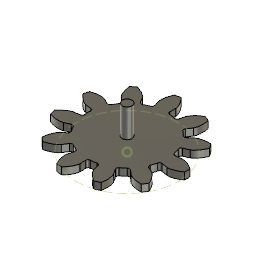
Slave gear (Autodesk Fusion 360 design; units mm, degrees)
description: Spur Gear; Module: 6.55; Num Teeth: 11; Pressure Angle: 20.0; Backlash: 0.00 mm
Autodesk Fusion 360 part; units mm, degrees
(part 1 of 3)
sketch "Sketch1" plane through (0, 0, 0) normal (0, 0, 1) x (1, 0, 0) in component "Spur Gear (11 teeth)"
  circle A0 centre (0, 0) radius 28.1142
extrude "Extrude1" add sketch "Sketch1" along normal blind 10 in component "Spur Gear (11 teeth)"
sketch "Sketch2" plane through (0, 0, 0) normal (0, 0, 1) x (1, 0, 0) in component "Spur Gear (11 teeth)"
  spline S0 degree 5 poles (33.4323, -5.3166) (33.4583, -5.3207) (33.5104, -5.3281) (33.5887, -5.3365) (33.6936, -5.3428) (33.8252, -5.344) (33.9572, -5.3403) (34.0895, -5.3337) (34.2219, -5.3256) (34.3544, -5.3164) (34.4869, -5.3059) (34.6196, -5.2938) (34.7523, -5.2796) (34.8851, -5.263) (35.018, -5.2439) (35.1509, -5.2227) (35.2838, -5.1996) (35.4168, -5.175) (35.5497, -5.149) (35.6826, -5.1217) (35.8155, -5.093) (35.9483, -5.0629) (36.0811, -5.0314) (36.2138, -4.9983) (36.3465, -4.9637) (36.4791, -4.9277) (36.6117, -4.8903) (36.7441, -4.8516) (36.8765, -4.8117) (37.0087, -4.7706) (37.1408, -4.7282) (37.2729, -4.6847) (37.4048, -4.6398) (37.5366, -4.5938) (37.6683, -4.5466) (37.7998, -4.4982) (37.9312, -4.4486) (38.0624, -4.3979) (38.1935, -4.3461) (38.3245, -4.2932) (38.4553, -4.2392) (38.5859, -4.1841) (38.7163, -4.1279) (38.8466, -4.0706) (38.9767, -4.0123) (39.1066, -3.9529) (39.2363, -3.8924) (39.3658, -3.831) (39.4951, -3.7685) (39.6243, -3.705) (39.7532, -3.6406) (39.8819, -3.5751) (40.0104, -3.5086) (40.1386, -3.4412) (40.2667, -3.3727) (40.3945, -3.3033) (40.5221, -3.233) (40.6494, -3.1617) (40.7765, -3.0895) (40.9034, -3.0163) (41.03, -2.9422) (41.1564, -2.8672) (41.2825, -2.7912) (41.4084, -2.7144) (41.534, -2.6366) (41.6593, -2.558) (41.7844, -2.4784) (41.9092, -2.398) (42.0337, -2.3167) (42.1579, -2.2345) (42.2818, -2.1514) (42.3808, -2.0843) (42.4548, -2.0335) (42.5042, -1.9995) (42.5288, -1.9825) knots 0 0 0 0 0 0 0.01428571 0.02857143 0.04285714 0.05714286 0.07142857 0.08571429 0.1 0.11428571 0.12857143 0.14285714 0.15714286 0.17142857 0.18571429 0.2 0.21428571 0.22857143 0.24285714 0.25714286 0.27142857 0.28571429 0.3 0.31428571 0.32857143 0.34285714 0.35714286 0.37142857 0.38571429 0.4 0.41428571 0.42857143 0.44285714 0.45714286 0.47142857 0.48571429 0.5 0.51428571 0.52857143 0.54285714 0.55714286 0.57142857 0.58571429 0.6 0.61428571 0.62857143 0.64285714 0.65714286 0.67142857 0.68571429 0.7 0.71428571 0.72857143 0.74285714 0.75714286 0.77142857 0.78571429 0.8 0.81428571 0.82857143 0.84285714 0.85714286 0.87142857 0.88571429 0.9 0.91428571 0.92857143 0.94285714 0.95714286 0.97142857 0.98571429 1 1 1 1 1 1
  spline S1 degree 5 poles (33.4323, 5.3166) (33.4583, 5.3207) (33.5104, 5.3281) (33.5887, 5.3365) (33.6936, 5.3428) (33.8252, 5.344) (33.9572, 5.3403) (34.0895, 5.3337) (34.2219, 5.3256) (34.3544, 5.3164) (34.4869, 5.3059) (34.6196, 5.2938) (34.7523, 5.2796) (34.8851, 5.263) (35.018, 5.2439) (35.1509, 5.2227) (35.2838, 5.1996) (35.4168, 5.175) (35.5497, 5.149) (35.6826, 5.1217) (35.8155, 5.093) (35.9483, 5.0629) (36.0811, 5.0314) (36.2138, 4.9983) (36.3465, 4.9637) (36.4791, 4.9277) (36.6117, 4.8903) (36.7441, 4.8516) (36.8765, 4.8117) (37.0087, 4.7706) (37.1408, 4.7282) (37.2729, 4.6847) (37.4048, 4.6398) (37.5366, 4.5938) (37.6683, 4.5466) (37.7998, 4.4982) (37.9312, 4.4486) (38.0624, 4.3979) (38.1935, 4.3461) (38.3245, 4.2932) (38.4553, 4.2392) (38.5859, 4.1841) (38.7163, 4.1279) (38.8466, 4.0706) (38.9767, 4.0123) (39.1066, 3.9529) (39.2363, 3.8924) (39.3658, 3.831) (39.4951, 3.7685) (39.6243, 3.705) (39.7532, 3.6406) (39.8819, 3.5751) (40.0104, 3.5086) (40.1386, 3.4412) (40.2667, 3.3727) (40.3945, 3.3033) (40.5221, 3.233) (40.6494, 3.1617) (40.7765, 3.0895) (40.9034, 3.0163) (41.03, 2.9422) (41.1564, 2.8672) (41.2825, 2.7912) (41.4084, 2.7144) (41.534, 2.6366) (41.6593, 2.558) (41.7844, 2.4784) (41.9092, 2.398) (42.0337, 2.3167) (42.1579, 2.2345) (42.2818, 2.1514) (42.3808, 2.0843) (42.4548, 2.0335) (42.5042, 1.9995) (42.5288, 1.9825) knots 0 0 0 0 0 0 0.01428571 0.02857143 0.04285714 0.05714286 0.07142857 0.08571429 0.1 0.11428571 0.12857143 0.14285714 0.15714286 0.17142857 0.18571429 0.2 0.21428571 0.22857143 0.24285714 0.25714286 0.27142857 0.28571429 0.3 0.31428571 0.32857143 0.34285714 0.35714286 0.37142857 0.38571429 0.4 0.41428571 0.42857143 0.44285714 0.45714286 0.47142857 0.48571429 0.5 0.51428571 0.52857143 0.54285714 0.55714286 0.57142857 0.58571429 0.6 0.61428571 0.62857143 0.64285714 0.65714286 0.67142857 0.68571429 0.7 0.71428571 0.72857143 0.74285714 0.75714286 0.77142857 0.78571429 0.8 0.81428571 0.82857143 0.84285714 0.85714286 0.87142857 0.88571429 0.9 0.91428571 0.92857143 0.94285714 0.95714286 0.97142857 0.98571429 1 1 1 1 1 1
  arc A0 (42.5288, -1.9825) -> (42.5288, 1.9825) centre (0, 0) ccw
  line L0 (27.7554, -4.4154) -> (33.4323, -5.3166)
  line L1 (27.7554, 4.4154) -> (33.4323, 5.3166)
  line L2 (27.7554, -4.4154) -> (27.7554, 4.4154)
  point P0 (34.0602, -5.3349)
  point P1 (34.6983, -5.2851)
  point P2 (35.3427, -5.1885)
  point P3 (35.9917, -5.0524)
  point P4 (36.644, -4.8806)
  point P5 (37.2988, -4.6757)
  point P6 (37.955, -4.4392)
  point P7 (38.612, -4.1726)
  point P8 (39.2689, -3.8768)
  point P9 (39.9251, -3.5526)
  point P10 (40.5799, -3.2005)
  point P11 (41.2325, -2.8212)
  point P12 (41.8824, -2.4151)
  point P13 (34.0602, 5.3349)
  point P14 (34.6983, 5.2851)
  point P15 (35.3427, 5.1885)
  point P16 (35.9917, 5.0524)
  point P17 (36.644, 4.8806)
  point P18 (37.2988, 4.6757)
  point P19 (37.955, 4.4392)
  point P20 (38.612, 4.1726)
  point P21 (39.2689, 3.8768)
  point P22 (39.9251, 3.5526)
  point P23 (40.5799, 3.2005)
  point P24 (41.2325, 2.8212)
  point P25 (41.8824, 2.4151)
extrude "Extrude2" add sketch "Sketch2" along normal blind 10 in component "Spur Gear (11 teeth)"
fillet "Fillet1" radius 1.5875 2 edges at (27.7651, -4.4169, 5) (27.7651, 4.4169, 5) in component "Spur Gear (11 teeth)"
pattern_circular "C-Pattern1" count 11 over 360 about axis through (0, 0, 0) along (0, 0, 1) of "Extrude2", "Fillet1" in component "Spur Gear (11 teeth)"
sketch "Sketch3" plane through (0, 0, 0) normal (0, 0, 1) x (1, 0, 0) in component "Spur Gear (11 teeth)"
  circle A0 centre (0, 0) radius 36.025 construction
sketch "Sketch1 (2)" plane through (0, 0, 10) normal (0, 0, 1) x (-1, 0, 0)
  arc A0 (-26.3122, 9.9035) -> (-27.4894, 5.8941) centre (0, 0) ccw
  arc A1 (-29.2905, 4.6591) -> (-27.4894, 5.8941) centre (-29.0416, 6.2269) ccw
  line L0 (-29.2905, 4.6591) -> (-33.4323, 5.3166)
  spline S0 degree 5 poles (-33.4323, 5.3166) (-33.4583, 5.3207) (-33.5104, 5.3281) (-33.5887, 5.3365) (-33.6936, 5.3428) (-33.8252, 5.344) (-33.9572, 5.3403) (-34.0895, 5.3337) (-34.2219, 5.3256) (-34.3544, 5.3164) (-34.4869, 5.3059) (-34.6196, 5.2938) (-34.7523, 5.2796) (-34.8851, 5.263) (-35.018, 5.2439) (-35.1509, 5.2227) (-35.2838, 5.1996) (-35.4168, 5.175) (-35.5497, 5.149) (-35.6826, 5.1217) (-35.8155, 5.093) (-35.9483, 5.0629) (-36.0811, 5.0314) (-36.2138, 4.9983) (-36.3465, 4.9637) (-36.4791, 4.9277) (-36.6117, 4.8903) (-36.7441, 4.8516) (-36.8765, 4.8117) (-37.0087, 4.7706) (-37.1408, 4.7282) (-37.2729, 4.6847) (-37.4048, 4.6398) (-37.5366, 4.5938) (-37.6683, 4.5466) (-37.7998, 4.4982) (-37.9312, 4.4486) (-38.0624, 4.3979) (-38.1935, 4.3461) (-38.3245, 4.2932) (-38.4553, 4.2392) (-38.5859, 4.1841) (-38.7163, 4.1279) (-38.8466, 4.0706) (-38.9767, 4.0123) (-39.1066, 3.9529) (-39.2363, 3.8924) (-39.3658, 3.831) (-39.4951, 3.7685) (-39.6243, 3.705) (-39.7532, 3.6406) (-39.8819, 3.5751) (-40.0104, 3.5086) (-40.1386, 3.4412) (-40.2667, 3.3727) (-40.3945, 3.3033) (-40.5221, 3.233) (-40.6494, 3.1617) (-40.7765, 3.0895) (-40.9034, 3.0163) (-41.03, 2.9422) (-41.1564, 2.8672) (-41.2825, 2.7912) (-41.4084, 2.7144) (-41.534, 2.6366) (-41.6593, 2.558) (-41.7844, 2.4784) (-41.9092, 2.398) (-42.0337, 2.3167) (-42.1579, 2.2345) (-42.2818, 2.1514) (-42.3808, 2.0843) (-42.4548, 2.0335) (-42.5042, 1.9995) (-42.5288, 1.9825) knots 0 0 0 0 0 0 0.01428571 0.02857143 0.04285714 0.05714286 0.07142857 0.08571429 0.1 0.11428571 0.12857143 0.14285714 0.15714286 0.17142857 0.18571429 0.2 0.21428571 0.22857143 0.24285714 0.25714286 0.27142857 0.28571429 0.3 0.31428571 0.32857143 0.34285714 0.35714286 0.37142857 0.38571429 0.4 0.41428571 0.42857143 0.44285714 0.45714286 0.47142857 0.48571429 0.5 0.51428571 0.52857143 0.54285714 0.55714286 0.57142857 0.58571429 0.6 0.61428571 0.62857143 0.64285714 0.65714286 0.67142857 0.68571429 0.7 0.71428571 0.72857143 0.74285714 0.75714286 0.77142857 0.78571429 0.8 0.81428571 0.82857143 0.84285714 0.85714286 0.87142857 0.88571429 0.9 0.91428571 0.92857143 0.94285714 0.95714286 0.97142857 0.98571429 1 1 1 1 1 1
  arc A2 (-42.5288, 1.9825) -> (-42.5288, -1.9825) centre (0, 0) ccw
  spline S1 degree 5 poles (-42.5288, -1.9825) (-42.5042, -1.9995) (-42.4548, -2.0335) (-42.3808, -2.0843) (-42.2818, -2.1514) (-42.1579, -2.2345) (-42.0337, -2.3167) (-41.9092, -2.398) (-41.7844, -2.4784) (-41.6593, -2.558) (-41.534, -2.6366) (-41.4084, -2.7144) (-41.2825, -2.7912) (-41.1564, -2.8672) (-41.03, -2.9422) (-40.9034, -3.0163) (-40.7765, -3.0895) (-40.6494, -3.1617) (-40.5221, -3.233) (-40.3945, -3.3033) (-40.2667, -3.3727) (-40.1386, -3.4412) (-40.0104, -3.5086) (-39.8819, -3.5751) (-39.7532, -3.6406) (-39.6243, -3.705) (-39.4951, -3.7685) (-39.3658, -3.831) (-39.2363, -3.8924) (-39.1066, -3.9529) (-38.9767, -4.0123) (-38.8466, -4.0706) (-38.7163, -4.1279) (-38.5859, -4.1841) (-38.4553, -4.2392) (-38.3245, -4.2932) (-38.1935, -4.3461) (-38.0624, -4.3979) (-37.9312, -4.4486) (-37.7998, -4.4982) (-37.6683, -4.5466) (-37.5366, -4.5938) (-37.4048, -4.6398) (-37.2729, -4.6847) (-37.1408, -4.7282) (-37.0087, -4.7706) (-36.8765, -4.8117) (-36.7441, -4.8516) (-36.6117, -4.8903) (-36.4791, -4.9277) (-36.3465, -4.9637) (-36.2138, -4.9983) (-36.0811, -5.0314) (-35.9483, -5.0629) (-35.8155, -5.093) (-35.6826, -5.1217) (-35.5497, -5.149) (-35.4168, -5.175) (-35.2838, -5.1996) (-35.1509, -5.2227) (-35.018, -5.2439) (-34.8851, -5.263) (-34.7523, -5.2796) (-34.6196, -5.2938) (-34.4869, -5.3059) (-34.3544, -5.3164) (-34.2219, -5.3256) (-34.0895, -5.3337) (-33.9572, -5.3403) (-33.8252, -5.344) (-33.6936, -5.3428) (-33.5887, -5.3365) (-33.5104, -5.3281) (-33.4583, -5.3207) (-33.4323, -5.3166) knots -1 -1 -1 -1 -1 -1 -0.98571429 -0.97142857 -0.95714286 -0.94285714 -0.92857143 -0.91428571 -0.9 -0.88571429 -0.87142857 -0.85714286 -0.84285714 -0.82857143 -0.81428571 -0.8 -0.78571429 -0.77142857 -0.75714286 -0.74285714 -0.72857143 -0.71428571 -0.7 -0.68571429 -0.67142857 -0.65714286 -0.64285714 -0.62857143 -0.61428571 -0.6 -0.58571429 -0.57142857 -0.55714286 -0.54285714 -0.52857143 -0.51428571 -0.5 -0.48571429 -0.47142857 -0.45714286 -0.44285714 -0.42857143 -0.41428571 -0.4 -0.38571429 -0.37142857 -0.35714286 -0.34285714 -0.32857143 -0.31428571 -0.3 -0.28571429 -0.27142857 -0.25714286 -0.24285714 -0.22857143 -0.21428571 -0.2 -0.18571429 -0.17142857 -0.15714286 -0.14285714 -0.12857143 -0.11428571 -0.1 -0.08571429 -0.07142857 -0.05714286 -0.04285714 -0.02857143 -0.01428571 0 0 0 0 0 0
  line L1 (-33.4323, -5.3166) -> (-29.2905, -4.6591)
  arc A3 (-27.4894, -5.8941) -> (-29.2905, -4.6591) centre (-29.0416, -6.2269) ccw
  arc A4 (-27.4894, -5.8941) -> (-26.3122, -9.9035) centre (0, 0) ccw
  arc A5 (-27.1596, -11.9162) -> (-26.3122, -9.9035) centre (-27.7979, -10.4627) ccw
  line L2 (-27.1596, -11.9162) -> (-30.9994, -13.6023)
  spline S2 degree 5 poles (-30.9994, -13.6023) (-31.0235, -13.6129) (-31.0713, -13.6348) (-31.1418, -13.6701) (-31.2334, -13.7214) (-31.3447, -13.7916) (-31.4538, -13.8661) (-31.5615, -13.9431) (-31.6685, -14.0216) (-31.775, -14.101) (-31.8808, -14.1814) (-31.9859, -14.2633) (-32.0898, -14.347) (-32.1926, -14.4328) (-32.2941, -14.5207) (-32.3944, -14.6104) (-32.4938, -14.7017) (-32.5923, -14.7943) (-32.6901, -14.888) (-32.7871, -14.9829) (-32.8834, -15.0788) (-32.9789, -15.1759) (-33.0735, -15.2743) (-33.1673, -15.3739) (-33.2602, -15.4747) (-33.3523, -15.5767) (-33.4436, -15.6798) (-33.5341, -15.7839) (-33.6239, -15.889) (-33.7129, -15.9951) (-33.8011, -16.1022) (-33.8887, -16.2103) (-33.9754, -16.3193) (-34.0614, -16.4292) (-34.1466, -16.5402) (-34.2311, -16.652) (-34.3149, -16.7647) (-34.3979, -16.8783) (-34.4801, -16.9928) (-34.5617, -17.1081) (-34.6425, -17.2243) (-34.7226, -17.3412) (-34.8019, -17.459) (-34.8805, -17.5777) (-34.9585, -17.6971) (-35.0356, -17.8172) (-35.1121, -17.9382) (-35.1878, -18.0599) (-35.2628, -18.1824) (-35.3371, -18.3056) (-35.4107, -18.4296) (-35.4836, -18.5542) (-35.5558, -18.6796) (-35.6272, -18.8057) (-35.6979, -18.9325) (-35.7679, -19.06) (-35.8372, -19.1881) (-35.9058, -19.3169) (-35.9737, -19.4464) (-36.0409, -19.5766) (-36.1073, -19.7074) (-36.1731, -19.8388) (-36.2381, -19.9709) (-36.3025, -20.1036) (-36.3661, -20.2369) (-36.429, -20.3708) (-36.4912, -20.5054) (-36.5527, -20.6405) (-36.6135, -20.7762) (-36.6735, -20.9125) (-36.7329, -21.0494) (-36.7798, -21.1594) (-36.8147, -21.2421) (-36.8378, -21.2974) (-36.8493, -21.325) knots 0 0 0 0 0 0 0.01428571 0.02857143 0.04285714 0.05714286 0.07142857 0.08571429 0.1 0.11428571 0.12857143 0.14285714 0.15714286 0.17142857 0.18571429 0.2 0.21428571 0.22857143 0.24285714 0.25714286 0.27142857 0.28571429 0.3 0.31428571 0.32857143 0.34285714 0.35714286 0.37142857 0.38571429 0.4 0.41428571 0.42857143 0.44285714 0.45714286 0.47142857 0.48571429 0.5 0.51428571 0.52857143 0.54285714 0.55714286 0.57142857 0.58571429 0.6 0.61428571 0.62857143 0.64285714 0.65714286 0.67142857 0.68571429 0.7 0.71428571 0.72857143 0.74285714 0.75714286 0.77142857 0.78571429 0.8 0.81428571 0.82857143 0.84285714 0.85714286 0.87142857 0.88571429 0.9 0.91428571 0.92857143 0.94285714 0.95714286 0.97142857 0.98571429 1 1 1 1 1 1
  arc A6 (-36.8493, -21.325) -> (-34.7057, -24.6606) centre (0, 0) ccw
  spline S3 degree 5 poles (-34.7057, -24.6606) (-34.6758, -24.6616) (-34.6159, -24.6635) (-34.5261, -24.6662) (-34.4066, -24.6692) (-34.2574, -24.672) (-34.1085, -24.674) (-33.9598, -24.6751) (-33.8113, -24.6753) (-33.6631, -24.6746) (-33.5151, -24.673) (-33.3674, -24.6705) (-33.22, -24.6672) (-33.0729, -24.6629) (-32.926, -24.6576) (-32.7794, -24.6515) (-32.6331, -24.6445) (-32.4871, -24.6365) (-32.3415, -24.6277) (-32.1961, -24.6179) (-32.0511, -24.6071) (-31.9063, -24.5955) (-31.762, -24.5829) (-31.6179, -24.5693) (-31.4743, -24.5548) (-31.331, -24.5394) (-31.188, -24.523) (-31.0454, -24.5056) (-30.9033, -24.4873) (-30.7615, -24.468) (-30.6201, -24.4477) (-30.4791, -24.4264) (-30.3385, -24.4042) (-30.1984, -24.3809) (-30.0588, -24.3567) (-29.9195, -24.3314) (-29.7808, -24.3052) (-29.6425, -24.2779) (-29.5046, -24.2496) (-29.3673, -24.2202) (-29.2305, -24.1898) (-29.0942, -24.1584) (-28.9584, -24.1258) (-28.8232, -24.0922) (-28.6886, -24.0575) (-28.5545, -24.0217) (-28.421, -23.9848) (-28.2881, -23.9468) (-28.1558, -23.9077) (-28.0241, -23.8675) (-27.8931, -23.8261) (-27.7628, -23.7835) (-27.6332, -23.7396) (-27.5044, -23.6944) (-27.3764, -23.6479) (-27.2492, -23.6001) (-27.1226, -23.5513) (-26.9967, -23.5013) (-26.8715, -23.4501) (-26.7472, -23.3976) (-26.6239, -23.3436) (-26.5018, -23.2878) (-26.3811, -23.23) (-26.2618, -23.1702) (-26.1437, -23.1087) (-26.0265, -23.0458) (-25.91, -22.9819) (-25.7942, -22.9172) (-25.6794, -22.8512) (-25.5664, -22.7829) (-25.4563, -22.7108) (-25.3715, -22.6488) (-25.3102, -22.5993) (-25.2704, -22.565) (-25.2507, -22.5475) knots -1 -1 -1 -1 -1 -1 -0.98571429 -0.97142857 -0.95714286 -0.94285714 -0.92857143 -0.91428571 -0.9 -0.88571429 -0.87142857 -0.85714286 -0.84285714 -0.82857143 -0.81428571 -0.8 -0.78571429 -0.77142857 -0.75714286 -0.74285714 -0.72857143 -0.71428571 -0.7 -0.68571429 -0.67142857 -0.65714286 -0.64285714 -0.62857143 -0.61428571 -0.6 -0.58571429 -0.57142857 -0.55714286 -0.54285714 -0.52857143 -0.51428571 -0.5 -0.48571429 -0.47142857 -0.45714286 -0.44285714 -0.42857143 -0.41428571 -0.4 -0.38571429 -0.37142857 -0.35714286 -0.34285714 -0.32857143 -0.31428571 -0.3 -0.28571429 -0.27142857 -0.25714286 -0.24285714 -0.22857143 -0.21428571 -0.2 -0.18571429 -0.17142857 -0.15714286 -0.14285714 -0.12857143 -0.11428571 -0.1 -0.08571429 -0.07142857 -0.05714286 -0.04285714 -0.02857143 -0.01428571 0 0 0 0 0 0
  line L3 (-25.2507, -22.5475) -> (-22.1219, -19.7551)
  arc A7 (-19.939, -19.8203) -> (-22.1219, -19.7551) centre (-21.0648, -20.9395) ccw
  arc A8 (-19.939, -19.8203) -> (-16.781, -22.5567) centre (0, 0) ccw
  arc A9 (-16.4058, -24.7082) -> (-16.781, -22.5567) centre (-17.7285, -23.8304) ccw
  line L4 (-16.4058, -24.7082) -> (-18.7244, -28.2025)
  spline S4 degree 5 poles (-18.7244, -28.2025) (-18.739, -28.2245) (-18.7673, -28.2688) (-18.8075, -28.3365) (-18.8568, -28.4292) (-18.9125, -28.5485) (-18.964, -28.6701) (-19.013, -28.7931) (-19.0606, -28.917) (-19.1072, -29.0413) (-19.1528, -29.1663) (-19.1969, -29.2919) (-19.2391, -29.4186) (-19.2791, -29.5463) (-19.317, -29.6751) (-19.3529, -29.8048) (-19.3872, -29.9353) (-19.42, -30.0665) (-19.4516, -30.1982) (-19.482, -30.3304) (-19.5111, -30.4632) (-19.5389, -30.5965) (-19.5653, -30.7304) (-19.5903, -30.8649) (-19.614, -31) (-19.6363, -31.1356) (-19.6574, -31.2716) (-19.6772, -31.4082) (-19.6959, -31.5451) (-19.7135, -31.6825) (-19.7298, -31.8203) (-19.745, -31.9585) (-19.7591, -32.0971) (-19.772, -32.2361) (-19.7837, -32.3755) (-19.7943, -32.5153) (-19.8038, -32.6554) (-19.8122, -32.7958) (-19.8195, -32.9366) (-19.8258, -33.0777) (-19.831, -33.2191) (-19.8351, -33.3608) (-19.8382, -33.5028) (-19.8402, -33.6451) (-19.8412, -33.7877) (-19.8411, -33.9305) (-19.84, -34.0736) (-19.8379, -34.217) (-19.8348, -34.3605) (-19.8307, -34.5044) (-19.8256, -34.6484) (-19.8195, -34.7927) (-19.8124, -34.9372) (-19.8044, -35.0819) (-19.7953, -35.2268) (-19.7853, -35.3719) (-19.7743, -35.5171) (-19.7624, -35.6626) (-19.7495, -35.8082) (-19.7356, -35.954) (-19.7208, -36.1) (-19.7051, -36.2461) (-19.6884, -36.3924) (-19.6707, -36.5388) (-19.6522, -36.6854) (-19.6327, -36.832) (-19.6123, -36.9788) (-19.591, -37.1258) (-19.5687, -37.2728) (-19.5456, -37.4199) (-19.5215, -37.5672) (-19.5015, -37.6851) (-19.4862, -37.7735) (-19.4757, -37.8325) (-19.4704, -37.862) knots 0 0 0 0 0 0 0.01428571 0.02857143 0.04285714 0.05714286 0.07142857 0.08571429 0.1 0.11428571 0.12857143 0.14285714 0.15714286 0.17142857 0.18571429 0.2 0.21428571 0.22857143 0.24285714 0.25714286 0.27142857 0.28571429 0.3 0.31428571 0.32857143 0.34285714 0.35714286 0.37142857 0.38571429 0.4 0.41428571 0.42857143 0.44285714 0.45714286 0.47142857 0.48571429 0.5 0.51428571 0.52857143 0.54285714 0.55714286 0.57142857 0.58571429 0.6 0.61428571 0.62857143 0.64285714 0.65714286 0.67142857 0.68571429 0.7 0.71428571 0.72857143 0.74285714 0.75714286 0.77142857 0.78571429 0.8 0.81428571 0.82857143 0.84285714 0.85714286 0.87142857 0.88571429 0.9 0.91428571 0.92857143 0.94285714 0.95714286 0.97142857 0.98571429 1 1 1 1 1 1
  arc A10 (-19.4704, -37.862) -> (-15.8638, -39.5091) centre (0, 0) ccw
  spline S5 degree 5 poles (-15.8638, -39.5091) (-15.838, -39.4938) (-15.7866, -39.463) (-15.7097, -39.4167) (-15.6075, -39.3546) (-15.4805, -39.2764) (-15.3541, -39.1975) (-15.2284, -39.1181) (-15.1034, -39.038) (-14.9791, -38.9573) (-14.8555, -38.8759) (-14.7326, -38.794) (-14.6104, -38.7114) (-14.4889, -38.6283) (-14.3682, -38.5445) (-14.2482, -38.4601) (-14.1289, -38.3751) (-14.0104, -38.2894) (-13.8926, -38.2032) (-13.7757, -38.1164) (-13.6594, -38.0289) (-13.544, -37.9409) (-13.4294, -37.8522) (-13.3155, -37.763) (-13.2025, -37.6731) (-13.0903, -37.5826) (-12.9789, -37.4915) (-12.8684, -37.3999) (-12.7587, -37.3076) (-12.6498, -37.2147) (-12.5418, -37.1212) (-12.4347, -37.0271) (-12.3285, -36.9324) (-12.2232, -36.8371) (-12.1188, -36.7411) (-12.0153, -36.6446) (-11.9128, -36.5475) (-11.8112, -36.4498) (-11.7106, -36.3514) (-11.6109, -36.2525) (-11.5122, -36.153) (-11.4146, -36.0528) (-11.318, -35.9521) (-11.2224, -35.8507) (-11.1279, -35.7487) (-11.0345, -35.6461) (-10.9421, -35.5429) (-10.8509, -35.439) (-10.7607, -35.3346) (-10.6716, -35.2296) (-10.5838, -35.1239) (-10.4972, -35.0176) (-10.412, -34.9106) (-10.3281, -34.803) (-10.2455, -34.6946) (-10.1643, -34.5857) (-10.0842, -34.4762) (-10.0053, -34.366) (-9.9277, -34.2553) (-9.8515, -34.144) (-9.777, -34.0319) (-9.7044, -33.9189) (-9.6341, -33.805) (-9.5661, -33.6902) (-9.5, -33.5746) (-9.4354, -33.4583) (-9.3719, -33.3416) (-9.3095, -33.2246) (-9.2486, -33.107) (-9.1904, -32.9884) (-9.1368, -32.8682) (-9.099, -32.7702) (-9.0741, -32.6955) (-9.0592, -32.6451) (-9.0522, -32.6197) knots -1 -1 -1 -1 -1 -1 -0.98571429 -0.97142857 -0.95714286 -0.94285714 -0.92857143 -0.91428571 -0.9 -0.88571429 -0.87142857 -0.85714286 -0.84285714 -0.82857143 -0.81428571 -0.8 -0.78571429 -0.77142857 -0.75714286 -0.74285714 -0.72857143 -0.71428571 -0.7 -0.68571429 -0.67142857 -0.65714286 -0.64285714 -0.62857143 -0.61428571 -0.6 -0.58571429 -0.57142857 -0.55714286 -0.54285714 -0.52857143 -0.51428571 -0.5 -0.48571429 -0.47142857 -0.45714286 -0.44285714 -0.42857143 -0.41428571 -0.4 -0.38571429 -0.37142857 -0.35714286 -0.34285714 -0.32857143 -0.31428571 -0.3 -0.28571429 -0.27142857 -0.25714286 -0.24285714 -0.22857143 -0.21428571 -0.2 -0.18571429 -0.17142857 -0.15714286 -0.14285714 -0.12857143 -0.11428571 -0.1 -0.08571429 -0.07142857 -0.05714286 -0.04285714 -0.02857143 -0.01428571 0 0 0 0 0 0
  line L5 (-9.0522, -32.6197) -> (-7.9297, -28.579)
  arc A11 (-6.058, -27.4537) -> (-7.9297, -28.579) centre (-6.4001, -29.004) ccw
  arc A12 (-6.058, -27.4537) -> (-1.922, -28.0484) centre (0, 0) ccw
  arc A13 (-0.4432, -29.6554) -> (-1.922, -28.0484) centre (-2.0305, -29.6322) ccw
  line L6 (-0.4432, -29.6554) -> (-0.5045, -33.8487)
  spline S6 degree 5 poles (-0.5045, -33.8487) (-0.5049, -33.875) (-0.5048, -33.9276) (-0.502, -34.0063) (-0.4934, -34.111) (-0.4758, -34.2414) (-0.4533, -34.3715) (-0.428, -34.5015) (-0.4011, -34.6315) (-0.3731, -34.7613) (-0.3439, -34.891) (-0.3131, -35.0206) (-0.2801, -35.1499) (-0.2447, -35.279) (-0.207, -35.4078) (-0.167, -35.5364) (-0.1253, -35.6647) (-0.082, -35.7928) (-0.0373, -35.9207) (0.0086, -36.0483) (0.0559, -36.1758) (0.1046, -36.303) (0.1547, -36.4299) (0.2064, -36.5566) (0.2595, -36.683) (0.314, -36.8091) (0.3699, -36.935) (0.427, -37.0606) (0.4853, -37.1859) (0.5449, -37.3109) (0.6056, -37.4357) (0.6675, -37.5602) (0.7306, -37.6844) (0.7949, -37.8083) (0.8604, -37.9319) (0.9271, -38.0552) (0.9948, -38.1782) (1.0637, -38.3009) (1.1336, -38.4233) (1.2047, -38.5454) (1.2767, -38.6671) (1.3499, -38.7886) (1.4241, -38.9097) (1.4993, -39.0305) (1.5755, -39.1509) (1.6528, -39.2711) (1.7311, -39.3909) (1.8103, -39.5103) (1.8906, -39.6295) (1.9718, -39.7482) (2.054, -39.8666) (2.1371, -39.9847) (2.2212, -40.1024) (2.3062, -40.2198) (2.3921, -40.3368) (2.479, -40.4535) (2.5668, -40.5697) (2.6555, -40.6856) (2.7451, -40.8012) (2.8356, -40.9163) (2.9269, -41.0311) (3.0192, -41.1455) (3.1123, -41.2596) (3.2063, -41.3732) (3.3011, -41.4865) (3.3968, -41.5993) (3.4933, -41.7118) (3.5907, -41.8239) (3.6889, -41.9355) (3.7879, -42.0468) (3.8878, -42.1576) (3.9683, -42.246) (4.0291, -42.3121) (4.0698, -42.3561) (4.0902, -42.3781) knots 0 0 0 0 0 0 0.01428571 0.02857143 0.04285714 0.05714286 0.07142857 0.08571429 0.1 0.11428571 0.12857143 0.14285714 0.15714286 0.17142857 0.18571429 0.2 0.21428571 0.22857143 0.24285714 0.25714286 0.27142857 0.28571429 0.3 0.31428571 0.32857143 0.34285714 0.35714286 0.37142857 0.38571429 0.4 0.41428571 0.42857143 0.44285714 0.45714286 0.47142857 0.48571429 0.5 0.51428571 0.52857143 0.54285714 0.55714286 0.57142857 0.58571429 0.6 0.61428571 0.62857143 0.64285714 0.65714286 0.67142857 0.68571429 0.7 0.71428571 0.72857143 0.74285714 0.75714286 0.77142857 0.78571429 0.8 0.81428571 0.82857143 0.84285714 0.85714286 0.87142857 0.88571429 0.9 0.91428571 0.92857143 0.94285714 0.95714286 0.97142857 0.98571429 1 1 1 1 1 1
  arc A14 (4.0902, -42.3781) -> (8.0148, -41.8138) centre (0, 0) ccw
  spline S7 degree 5 poles (8.0148, -41.8138) (8.0282, -41.787) (8.0548, -41.7333) (8.0945, -41.6528) (8.1469, -41.5453) (8.2114, -41.4108) (8.2751, -41.2761) (8.3379, -41.1413) (8.3997, -41.0064) (8.4607, -40.8712) (8.5207, -40.736) (8.5798, -40.6006) (8.6379, -40.4651) (8.6952, -40.3295) (8.7514, -40.1937) (8.8068, -40.0578) (8.8611, -39.9218) (8.9145, -39.7857) (8.967, -39.6495) (9.0185, -39.5132) (9.0689, -39.3768) (9.1185, -39.2404) (9.167, -39.1038) (9.2145, -38.9672) (9.261, -38.8304) (9.3064, -38.6937) (9.3509, -38.5568) (9.3943, -38.4199) (9.4367, -38.283) (9.4781, -38.146) (9.5184, -38.0089) (9.5576, -37.8719) (9.5957, -37.7348) (9.6328, -37.5977) (9.6688, -37.4605) (9.7036, -37.3234) (9.7374, -37.1863) (9.77, -37.0491) (9.8015, -36.912) (9.8319, -36.7749) (9.8611, -36.6378) (9.8891, -36.5008) (9.9159, -36.3638) (9.9415, -36.2268) (9.9658, -36.0899) (9.9889, -35.9531) (10.0108, -35.8163) (10.0315, -35.6796) (10.0509, -35.543) (10.069, -35.4065) (10.0858, -35.2702) (10.1011, -35.1339) (10.115, -34.9978) (10.1274, -34.8619) (10.1383, -34.7261) (10.1477, -34.5905) (10.1558, -34.4551) (10.1627, -34.3198) (10.1681, -34.1847) (10.172, -34.0498) (10.1741, -33.9152) (10.174, -33.781) (10.1716, -33.6472) (10.1668, -33.5138) (10.1599, -33.3808) (10.1514, -33.2481) (10.1417, -33.1156) (10.1309, -32.9834) (10.1186, -32.8515) (10.1034, -32.7203) (10.0835, -32.5902) (10.0624, -32.4874) (10.0429, -32.411) (10.0282, -32.3606) (10.0204, -32.3354) knots -1 -1 -1 -1 -1 -1 -0.98571429 -0.97142857 -0.95714286 -0.94285714 -0.92857143 -0.91428571 -0.9 -0.88571429 -0.87142857 -0.85714286 -0.84285714 -0.82857143 -0.81428571 -0.8 -0.78571429 -0.77142857 -0.75714286 -0.74285714 -0.72857143 -0.71428571 -0.7 -0.68571429 -0.67142857 -0.65714286 -0.64285714 -0.62857143 -0.61428571 -0.6 -0.58571429 -0.57142857 -0.55714286 -0.54285714 -0.52857143 -0.51428571 -0.5 -0.48571429 -0.47142857 -0.45714286 -0.44285714 -0.42857143 -0.41428571 -0.4 -0.38571429 -0.37142857 -0.35714286 -0.34285714 -0.32857143 -0.31428571 -0.3 -0.28571429 -0.27142857 -0.25714286 -0.24285714 -0.22857143 -0.21428571 -0.2 -0.18571429 -0.17142857 -0.15714286 -0.14285714 -0.12857143 -0.11428571 -0.1 -0.08571429 -0.07142857 -0.05714286 -0.04285714 -0.02857143 -0.01428571 0 0 0 0 0 0
  line L7 (10.0204, -32.3354) -> (8.7801, -28.3293)
  arc A15 (9.7463, -26.3708) -> (8.7801, -28.3293) centre (10.2966, -27.8598) ccw
  arc A16 (9.7463, -26.3708) -> (13.5473, -24.6349) centre (0, 0) ccw
  arc A17 (15.6601, -25.1873) -> (13.5473, -24.6349) centre (14.3122, -26.026) ccw
  line L8 (15.6601, -25.1873) -> (17.8755, -28.7481)
  spline S8 degree 5 poles (17.8755, -28.7481) (17.8894, -28.7704) (17.918, -28.8146) (17.9629, -28.8793) (18.0267, -28.9627) (18.1121, -29.0629) (18.2013, -29.1603) (18.2929, -29.2559) (18.3857, -29.3507) (18.4795, -29.4448) (18.5742, -29.5381) (18.6702, -29.6304) (18.7678, -29.7214) (18.8674, -29.8109) (18.9688, -29.8988) (19.0719, -29.9854) (19.1764, -30.0708) (19.2821, -30.1551) (19.3888, -30.2386) (19.4964, -30.3211) (19.6051, -30.4028) (19.7148, -30.4835) (19.8257, -30.5631) (19.9376, -30.6418) (20.0506, -30.7194) (20.1647, -30.796) (20.2797, -30.8717) (20.3957, -30.9465) (20.5125, -31.0204) (20.6302, -31.0934) (20.7487, -31.1655) (20.8681, -31.2368) (20.9884, -31.3071) (21.1095, -31.3766) (21.2314, -31.4452) (21.3541, -31.5129) (21.4776, -31.5797) (21.6019, -31.6457) (21.7269, -31.7108) (21.8526, -31.7751) (21.9791, -31.8386) (22.1063, -31.9012) (22.2342, -31.963) (22.3628, -32.024) (22.492, -32.0841) (22.622, -32.1434) (22.7526, -32.2018) (22.8839, -32.2595) (23.0158, -32.3163) (23.1483, -32.3723) (23.2814, -32.4275) (23.4152, -32.4819) (23.5496, -32.5355) (23.6846, -32.5882) (23.8201, -32.6402) (23.9563, -32.6914) (24.093, -32.7417) (24.2303, -32.7913) (24.3681, -32.84) (24.5065, -32.888) (24.6454, -32.9352) (24.7849, -32.9815) (24.9248, -33.0271) (25.0653, -33.0719) (25.2064, -33.1159) (25.3479, -33.1591) (25.4899, -33.2015) (25.6324, -33.2432) (25.7754, -33.284) (25.9188, -33.3241) (26.0628, -33.3634) (26.1783, -33.3942) (26.2652, -33.4169) (26.3232, -33.4319) (26.3522, -33.4394) knots 0 0 0 0 0 0 0.01428571 0.02857143 0.04285714 0.05714286 0.07142857 0.08571429 0.1 0.11428571 0.12857143 0.14285714 0.15714286 0.17142857 0.18571429 0.2 0.21428571 0.22857143 0.24285714 0.25714286 0.27142857 0.28571429 0.3 0.31428571 0.32857143 0.34285714 0.35714286 0.37142857 0.38571429 0.4 0.41428571 0.42857143 0.44285714 0.45714286 0.47142857 0.48571429 0.5 0.51428571 0.52857143 0.54285714 0.55714286 0.57142857 0.58571429 0.6 0.61428571 0.62857143 0.64285714 0.65714286 0.67142857 0.68571429 0.7 0.71428571 0.72857143 0.74285714 0.75714286 0.77142857 0.78571429 0.8 0.81428571 0.82857143 0.84285714 0.85714286 0.87142857 0.88571429 0.9 0.91428571 0.92857143 0.94285714 0.95714286 0.97142857 0.98571429 1 1 1 1 1 1
  arc A18 (26.3522, -33.4394) -> (29.3487, -30.8429) centre (0, 0) ccw
  spline S9 degree 5 poles (29.3487, -30.8429) (29.3455, -30.8131) (29.3389, -30.7535) (29.3287, -30.6643) (29.3147, -30.5456) (29.2963, -30.3975) (29.277, -30.2498) (29.2569, -30.1025) (29.236, -29.9555) (29.2142, -29.8089) (29.1916, -29.6627) (29.1681, -29.5168) (29.1438, -29.3714) (29.1186, -29.2263) (29.0925, -29.0817) (29.0656, -28.9375) (29.0378, -28.7937) (29.0092, -28.6503) (28.9797, -28.5074) (28.9493, -28.3649) (28.918, -28.2229) (28.8859, -28.0813) (28.8528, -27.9402) (28.8189, -27.7995) (28.7841, -27.6594) (28.7485, -27.5197) (28.7119, -27.3806) (28.6744, -27.2419) (28.636, -27.1038) (28.5967, -26.9662) (28.5566, -26.8291) (28.5154, -26.6926) (28.4734, -26.5567) (28.4305, -26.4213) (28.3866, -26.2865) (28.3418, -26.1523) (28.296, -26.0186) (28.2493, -25.8856) (28.2017, -25.7532) (28.1531, -25.6215) (28.1036, -25.4904) (28.053, -25.3599) (28.0015, -25.2302) (27.949, -25.1012) (27.8954, -24.9728) (27.8409, -24.8452) (27.7854, -24.7184) (27.7289, -24.5922) (27.6714, -24.4668) (27.6128, -24.3422) (27.5532, -24.2184) (27.4925, -24.0954) (27.4305, -23.9734) (27.3675, -23.8524) (27.3032, -23.7323) (27.2379, -23.6131) (27.1715, -23.4948) (27.1041, -23.3773) (27.0356, -23.2607) (26.966, -23.1451) (26.895, -23.0308) (26.8223, -22.9179) (26.748, -22.8066) (26.6718, -22.697) (26.5941, -22.5889) (26.5152, -22.4818) (26.4354, -22.3756) (26.3548, -22.2702) (26.2732, -22.166) (26.1895, -22.0638) (26.1024, -21.9651) (26.029, -21.89) (25.9713, -21.8363) (25.9317, -21.8018) (25.9115, -21.7849) knots -1 -1 -1 -1 -1 -1 -0.98571429 -0.97142857 -0.95714286 -0.94285714 -0.92857143 -0.91428571 -0.9 -0.88571429 -0.87142857 -0.85714286 -0.84285714 -0.82857143 -0.81428571 -0.8 -0.78571429 -0.77142857 -0.75714286 -0.74285714 -0.72857143 -0.71428571 -0.7 -0.68571429 -0.67142857 -0.65714286 -0.64285714 -0.62857143 -0.61428571 -0.6 -0.58571429 -0.57142857 -0.55714286 -0.54285714 -0.52857143 -0.51428571 -0.5 -0.48571429 -0.47142857 -0.45714286 -0.44285714 -0.42857143 -0.41428571 -0.4 -0.38571429 -0.37142857 -0.35714286 -0.34285714 -0.32857143 -0.31428571 -0.3 -0.28571429 -0.27142857 -0.25714286 -0.24285714 -0.22857143 -0.21428571 -0.2 -0.18571429 -0.17142857 -0.15714286 -0.14285714 -0.12857143 -0.11428571 -0.1 -0.08571429 -0.07142857 -0.05714286 -0.04285714 -0.02857143 -0.01428571 0 0 0 0 0 0
  line L9 (25.9115, -21.7849) -> (22.7023, -19.0853)
  arc A19 (22.4562, -16.9153) -> (22.7023, -19.0853) centre (23.7242, -17.8704) ccw
  arc A20 (22.4562, -16.9153) -> (24.7153, -13.4) centre (0, 0) ccw
  arc A21 (26.7914, -12.7224) -> (24.7153, -13.4) centre (26.1109, -14.1567) ccw
  line L10 (26.7914, -12.7224) -> (30.5802, -14.5202)
  spline S10 degree 5 poles (30.5802, -14.5202) (30.604, -14.5315) (30.6519, -14.5532) (30.7247, -14.5834) (30.8235, -14.619) (30.9494, -14.6571) (31.0771, -14.6908) (31.2059, -14.7218) (31.3352, -14.7513) (31.465, -14.7798) (31.5951, -14.8071) (31.7258, -14.8328) (31.8571, -14.8566) (31.9892, -14.878) (32.1221, -14.8972) (32.2556, -14.9143) (32.3897, -14.9296) (32.5242, -14.9434) (32.6591, -14.956) (32.7943, -14.9672) (32.9299, -14.9771) (33.0658, -14.9857) (33.2021, -14.9928) (33.3388, -14.9984) (33.4758, -15.0026) (33.6132, -15.0054) (33.7509, -15.0069) (33.8888, -15.0071) (34.0271, -15.0061) (34.1656, -15.0039) (34.3043, -15.0005) (34.4432, -14.9959) (34.5824, -14.9901) (34.7219, -14.983) (34.8615, -14.9748) (35.0013, -14.9654) (35.1414, -14.9549) (35.2816, -14.9432) (35.422, -14.9304) (35.5625, -14.9165) (35.7032, -14.9015) (35.8441, -14.8855) (35.9851, -14.8683) (36.1262, -14.85) (36.2675, -14.8307) (36.4088, -14.8103) (36.5503, -14.7889) (36.6919, -14.7664) (36.8336, -14.7429) (36.9754, -14.7184) (37.1172, -14.6928) (37.2592, -14.6663) (37.4012, -14.6387) (37.5433, -14.6101) (37.6854, -14.5805) (37.8276, -14.55) (37.9698, -14.5184) (38.1121, -14.4859) (38.2544, -14.4524) (38.3967, -14.4179) (38.5391, -14.3825) (38.6815, -14.3461) (38.8239, -14.3088) (38.9663, -14.2705) (39.1087, -14.2313) (39.2512, -14.1911) (39.3936, -14.15) (39.536, -14.108) (39.6783, -14.0651) (39.8207, -14.0212) (39.963, -13.9765) (40.0768, -13.9399) (40.1622, -13.9121) (40.2191, -13.8934) (40.2476, -13.8839) knots 0 0 0 0 0 0 0.01428571 0.02857143 0.04285714 0.05714286 0.07142857 0.08571429 0.1 0.11428571 0.12857143 0.14285714 0.15714286 0.17142857 0.18571429 0.2 0.21428571 0.22857143 0.24285714 0.25714286 0.27142857 0.28571429 0.3 0.31428571 0.32857143 0.34285714 0.35714286 0.37142857 0.38571429 0.4 0.41428571 0.42857143 0.44285714 0.45714286 0.47142857 0.48571429 0.5 0.51428571 0.52857143 0.54285714 0.55714286 0.57142857 0.58571429 0.6 0.61428571 0.62857143 0.64285714 0.65714286 0.67142857 0.68571429 0.7 0.71428571 0.72857143 0.74285714 0.75714286 0.77142857 0.78571429 0.8 0.81428571 0.82857143 0.84285714 0.85714286 0.87142857 0.88571429 0.9 0.91428571 0.92857143 0.94285714 0.95714286 0.97142857 0.98571429 1 1 1 1 1 1
  arc A22 (40.2476, -13.8839) -> (41.3646, -10.0796) centre (0, 0) ccw
  spline S11 degree 5 poles (41.3646, -10.0796) (41.3458, -10.0563) (41.308, -10.0097) (41.2513, -9.9402) (41.1753, -9.8479) (41.0797, -9.7333) (40.9837, -9.6194) (40.8871, -9.5063) (40.7901, -9.394) (40.6925, -9.2824) (40.5944, -9.1717) (40.4958, -9.0617) (40.3967, -8.9525) (40.2971, -8.8441) (40.1969, -8.7365) (40.0963, -8.6297) (39.9952, -8.5238) (39.8936, -8.4186) (39.7915, -8.3143) (39.6889, -8.2109) (39.5858, -8.1083) (39.4822, -8.0066) (39.3782, -7.9057) (39.2736, -7.8058) (39.1686, -7.7067) (39.063, -7.6085) (38.957, -7.5112) (38.8505, -7.4148) (38.7436, -7.3194) (38.6361, -7.2248) (38.5282, -7.1313) (38.4198, -7.0386) (38.311, -6.947) (38.2017, -6.8563) (38.0919, -6.7666) (37.9816, -6.678) (37.8709, -6.5903) (37.7597, -6.5036) (37.648, -6.418) (37.5359, -6.3334) (37.4234, -6.2499) (37.3103, -6.1675) (37.1968, -6.0862) (37.0829, -6.0061) (36.9685, -5.9271) (36.8536, -5.8492) (36.7383, -5.7725) (36.6226, -5.6969) (36.5064, -5.6225) (36.3897, -5.5493) (36.2727, -5.4774) (36.1551, -5.4068) (36.0371, -5.3377) (35.9186, -5.27) (35.7996, -5.2037) (35.6802, -5.1387) (35.5604, -5.0751) (35.4401, -5.0127) (35.3195, -4.9516) (35.1984, -4.892) (35.0769, -4.8342) (34.9547, -4.7785) (34.832, -4.7251) (34.7087, -4.6741) (34.5848, -4.6251) (34.4606, -4.5777) (34.336, -4.5315) (34.2113, -4.4864) (34.0862, -4.4429) (33.9606, -4.4021) (33.834, -4.3662) (33.7316, -4.3427) (33.6541, -4.3287) (33.602, -4.3211) (33.5759, -4.3178) knots -1 -1 -1 -1 -1 -1 -0.98571429 -0.97142857 -0.95714286 -0.94285714 -0.92857143 -0.91428571 -0.9 -0.88571429 -0.87142857 -0.85714286 -0.84285714 -0.82857143 -0.81428571 -0.8 -0.78571429 -0.77142857 -0.75714286 -0.74285714 -0.72857143 -0.71428571 -0.7 -0.68571429 -0.67142857 -0.65714286 -0.64285714 -0.62857143 -0.61428571 -0.6 -0.58571429 -0.57142857 -0.55714286 -0.54285714 -0.52857143 -0.51428571 -0.5 -0.48571429 -0.47142857 -0.45714286 -0.44285714 -0.42857143 -0.41428571 -0.4 -0.38571429 -0.37142857 -0.35714286 -0.34285714 -0.32857143 -0.31428571 -0.3 -0.28571429 -0.27142857 -0.25714286 -0.24285714 -0.22857143 -0.21428571 -0.2 -0.18571429 -0.17142857 -0.15714286 -0.14285714 -0.12857143 -0.11428571 -0.1 -0.08571429 -0.07142857 -0.05714286 -0.04285714 -0.02857143 -0.01428571 0 0 0 0 0 0
  line L11 (33.5759, -4.3178) -> (29.4167, -3.7818)
  arc A23 (28.0365, -2.0893) -> (29.4167, -3.7818) centre (29.6196, -2.2073) ccw
  arc A24 (28.0365, -2.0893) -> (28.0365, 2.0893) centre (0, 0) ccw
  arc A25 (29.4167, 3.7818) -> (28.0365, 2.0893) centre (29.6196, 2.2073) ccw
  line L12 (29.4167, 3.7818) -> (33.5759, 4.3178)
  spline S12 degree 5 poles (33.5759, 4.3178) (33.602, 4.3211) (33.6541, 4.3287) (33.7316, 4.3427) (33.834, 4.3662) (33.9606, 4.4021) (34.0862, 4.4429) (34.2113, 4.4864) (34.336, 4.5315) (34.4606, 4.5777) (34.5848, 4.6251) (34.7087, 4.6741) (34.832, 4.7251) (34.9547, 4.7785) (35.0769, 4.8342) (35.1984, 4.892) (35.3195, 4.9516) (35.4401, 5.0127) (35.5604, 5.0751) (35.6802, 5.1387) (35.7996, 5.2037) (35.9186, 5.27) (36.0371, 5.3377) (36.1551, 5.4068) (36.2727, 5.4774) (36.3897, 5.5493) (36.5064, 5.6225) (36.6226, 5.6969) (36.7383, 5.7725) (36.8536, 5.8492) (36.9685, 5.9271) (37.0829, 6.0061) (37.1968, 6.0862) (37.3103, 6.1675) (37.4234, 6.2499) (37.5359, 6.3334) (37.648, 6.418) (37.7597, 6.5036) (37.8709, 6.5903) (37.9816, 6.678) (38.0919, 6.7666) (38.2017, 6.8563) (38.311, 6.947) (38.4198, 7.0386) (38.5282, 7.1313) (38.6361, 7.2248) (38.7436, 7.3194) (38.8505, 7.4148) (38.957, 7.5112) (39.063, 7.6085) (39.1686, 7.7067) (39.2736, 7.8058) (39.3782, 7.9057) (39.4822, 8.0066) (39.5858, 8.1083) (39.6889, 8.2109) (39.7915, 8.3143) (39.8936, 8.4186) (39.9952, 8.5238) (40.0963, 8.6297) (40.1969, 8.7365) (40.2971, 8.8441) (40.3967, 8.9525) (40.4958, 9.0617) (40.5944, 9.1717) (40.6925, 9.2824) (40.7901, 9.394) (40.8871, 9.5063) (40.9837, 9.6194) (41.0797, 9.7333) (41.1753, 9.8479) (41.2513, 9.9402) (41.308, 10.0097) (41.3458, 10.0563) (41.3646, 10.0796) knots 0 0 0 0 0 0 0.01428571 0.02857143 0.04285714 0.05714286 0.07142857 0.08571429 0.1 0.11428571 0.12857143 0.14285714 0.15714286 0.17142857 0.18571429 0.2 0.21428571 0.22857143 0.24285714 0.25714286 0.27142857 0.28571429 0.3 0.31428571 0.32857143 0.34285714 0.35714286 0.37142857 0.38571429 0.4 0.41428571 0.42857143 0.44285714 0.45714286 0.47142857 0.48571429 0.5 0.51428571 0.52857143 0.54285714 0.55714286 0.57142857 0.58571429 0.6 0.61428571 0.62857143 0.64285714 0.65714286 0.67142857 0.68571429 0.7 0.71428571 0.72857143 0.74285714 0.75714286 0.77142857 0.78571429 0.8 0.81428571 0.82857143 0.84285714 0.85714286 0.87142857 0.88571429 0.9 0.91428571 0.92857143 0.94285714 0.95714286 0.97142857 0.98571429 1 1 1 1 1 1
  arc A26 (41.3646, 10.0796) -> (40.2476, 13.8839) centre (0, 0) ccw
  spline S13 degree 5 poles (40.2476, 13.8839) (40.2191, 13.8934) (40.1622, 13.9121) (40.0768, 13.9399) (39.963, 13.9765) (39.8207, 14.0212) (39.6783, 14.0651) (39.536, 14.108) (39.3936, 14.15) (39.2512, 14.1911) (39.1087, 14.2313) (38.9663, 14.2705) (38.8239, 14.3088) (38.6815, 14.3461) (38.5391, 14.3825) (38.3967, 14.4179) (38.2544, 14.4524) (38.1121, 14.4859) (37.9698, 14.5184) (37.8276, 14.55) (37.6854, 14.5805) (37.5433, 14.6101) (37.4012, 14.6387) (37.2592, 14.6663) (37.1172, 14.6928) (36.9754, 14.7184) (36.8336, 14.7429) (36.6919, 14.7664) (36.5503, 14.7889) (36.4088, 14.8103) (36.2675, 14.8307) (36.1262, 14.85) (35.9851, 14.8683) (35.8441, 14.8855) (35.7032, 14.9015) (35.5625, 14.9165) (35.422, 14.9304) (35.2816, 14.9432) (35.1414, 14.9549) (35.0013, 14.9654) (34.8615, 14.9748) (34.7219, 14.983) (34.5824, 14.9901) (34.4432, 14.9959) (34.3043, 15.0005) (34.1656, 15.0039) (34.0271, 15.0061) (33.8888, 15.0071) (33.7509, 15.0069) (33.6132, 15.0054) (33.4758, 15.0026) (33.3388, 14.9984) (33.2021, 14.9928) (33.0658, 14.9857) (32.9299, 14.9771) (32.7943, 14.9672) (32.6591, 14.956) (32.5242, 14.9434) (32.3897, 14.9296) (32.2556, 14.9143) (32.1221, 14.8972) (31.9892, 14.878) (31.8571, 14.8566) (31.7258, 14.8328) (31.5951, 14.8071) (31.465, 14.7798) (31.3352, 14.7513) (31.2059, 14.7218) (31.0771, 14.6908) (30.9494, 14.6571) (30.8235, 14.619) (30.7247, 14.5834) (30.6519, 14.5532) (30.604, 14.5315) (30.5802, 14.5202) knots -1 -1 -1 -1 -1 -1 -0.98571429 -0.97142857 -0.95714286 -0.94285714 -0.92857143 -0.91428571 -0.9 -0.88571429 -0.87142857 -0.85714286 -0.84285714 -0.82857143 -0.81428571 -0.8 -0.78571429 -0.77142857 -0.75714286 -0.74285714 -0.72857143 -0.71428571 -0.7 -0.68571429 -0.67142857 -0.65714286 -0.64285714 -0.62857143 -0.61428571 -0.6 -0.58571429 -0.57142857 -0.55714286 -0.54285714 -0.52857143 -0.51428571 -0.5 -0.48571429 -0.47142857 -0.45714286 -0.44285714 -0.42857143 -0.41428571 -0.4 -0.38571429 -0.37142857 -0.35714286 -0.34285714 -0.32857143 -0.31428571 -0.3 -0.28571429 -0.27142857 -0.25714286 -0.24285714 -0.22857143 -0.21428571 -0.2 -0.18571429 -0.17142857 -0.15714286 -0.14285714 -0.12857143 -0.11428571 -0.1 -0.08571429 -0.07142857 -0.05714286 -0.04285714 -0.02857143 -0.01428571 0 0 0 0 0 0
  line L13 (30.5802, 14.5202) -> (26.7914, 12.7224)
  arc A27 (24.7153, 13.4) -> (26.7914, 12.7224) centre (26.1109, 14.1567) ccw
  arc A28 (24.7153, 13.4) -> (22.4562, 16.9153) centre (0, 0) ccw
  arc A29 (22.7023, 19.0853) -> (22.4562, 16.9153) centre (23.7242, 17.8704) ccw
  line L14 (22.7023, 19.0853) -> (25.9115, 21.7849)
  spline S14 degree 5 poles (25.9115, 21.7849) (25.9317, 21.8018) (25.9713, 21.8363) (26.029, 21.89) (26.1024, 21.9651) (26.1895, 22.0638) (26.2732, 22.166) (26.3548, 22.2702) (26.4354, 22.3756) (26.5152, 22.4818) (26.5941, 22.5889) (26.6718, 22.697) (26.748, 22.8066) (26.8223, 22.9179) (26.895, 23.0308) (26.966, 23.1451) (27.0356, 23.2607) (27.1041, 23.3773) (27.1715, 23.4948) (27.2379, 23.6131) (27.3032, 23.7323) (27.3675, 23.8524) (27.4305, 23.9734) (27.4925, 24.0954) (27.5532, 24.2184) (27.6128, 24.3422) (27.6714, 24.4668) (27.7289, 24.5922) (27.7854, 24.7184) (27.8409, 24.8452) (27.8954, 24.9728) (27.949, 25.1012) (28.0015, 25.2302) (28.053, 25.3599) (28.1036, 25.4904) (28.1531, 25.6215) (28.2017, 25.7532) (28.2493, 25.8856) (28.296, 26.0186) (28.3418, 26.1523) (28.3866, 26.2865) (28.4305, 26.4213) (28.4734, 26.5567) (28.5154, 26.6926) (28.5566, 26.8291) (28.5967, 26.9662) (28.636, 27.1038) (28.6744, 27.2419) (28.7119, 27.3806) (28.7485, 27.5197) (28.7841, 27.6594) (28.8189, 27.7995) (28.8528, 27.9402) (28.8859, 28.0813) (28.918, 28.2229) (28.9493, 28.3649) (28.9797, 28.5074) (29.0092, 28.6503) (29.0378, 28.7937) (29.0656, 28.9375) (29.0925, 29.0817) (29.1186, 29.2263) (29.1438, 29.3714) (29.1681, 29.5168) (29.1916, 29.6627) (29.2142, 29.8089) (29.236, 29.9555) (29.2569, 30.1025) (29.277, 30.2498) (29.2963, 30.3975) (29.3147, 30.5456) (29.3287, 30.6643) (29.3389, 30.7535) (29.3455, 30.8131) (29.3487, 30.8429) knots 0 0 0 0 0 0 0.01428571 0.02857143 0.04285714 0.05714286 0.07142857 0.08571429 0.1 0.11428571 0.12857143 0.14285714 0.15714286 0.17142857 0.18571429 0.2 0.21428571 0.22857143 0.24285714 0.25714286 0.27142857 0.28571429 0.3 0.31428571 0.32857143 0.34285714 0.35714286 0.37142857 0.38571429 0.4 0.41428571 0.42857143 0.44285714 0.45714286 0.47142857 0.48571429 0.5 0.51428571 0.52857143 0.54285714 0.55714286 0.57142857 0.58571429 0.6 0.61428571 0.62857143 0.64285714 0.65714286 0.67142857 0.68571429 0.7 0.71428571 0.72857143 0.74285714 0.75714286 0.77142857 0.78571429 0.8 0.81428571 0.82857143 0.84285714 0.85714286 0.87142857 0.88571429 0.9 0.91428571 0.92857143 0.94285714 0.95714286 0.97142857 0.98571429 1 1 1 1 1 1
  arc A30 (29.3487, 30.8429) -> (26.3522, 33.4394) centre (0, 0) ccw
  spline S15 degree 5 poles (26.3522, 33.4394) (26.3232, 33.4319) (26.2652, 33.4169) (26.1783, 33.3942) (26.0628, 33.3634) (25.9188, 33.3241) (25.7754, 33.284) (25.6324, 33.2432) (25.4899, 33.2015) (25.3479, 33.1591) (25.2064, 33.1159) (25.0653, 33.0719) (24.9248, 33.0271) (24.7849, 32.9815) (24.6454, 32.9352) (24.5065, 32.888) (24.3681, 32.84) (24.2303, 32.7913) (24.093, 32.7417) (23.9563, 32.6914) (23.8201, 32.6402) (23.6846, 32.5882) (23.5496, 32.5355) (23.4152, 32.4819) (23.2814, 32.4275) (23.1483, 32.3723) (23.0158, 32.3163) (22.8839, 32.2595) (22.7526, 32.2018) (22.622, 32.1434) (22.492, 32.0841) (22.3628, 32.024) (22.2342, 31.963) (22.1063, 31.9012) (21.9791, 31.8386) (21.8526, 31.7751) (21.7269, 31.7108) (21.6019, 31.6457) (21.4776, 31.5797) (21.3541, 31.5129) (21.2314, 31.4452) (21.1095, 31.3766) (20.9884, 31.3071) (20.8681, 31.2368) (20.7487, 31.1655) (20.6302, 31.0934) (20.5125, 31.0204) (20.3957, 30.9465) (20.2797, 30.8717) (20.1647, 30.796) (20.0506, 30.7194) (19.9376, 30.6418) (19.8257, 30.5631) (19.7148, 30.4835) (19.6051, 30.4028) (19.4964, 30.3211) (19.3888, 30.2386) (19.2821, 30.1551) (19.1764, 30.0708) (19.0719, 29.9854) (18.9688, 29.8988) (18.8674, 29.8109) (18.7678, 29.7214) (18.6702, 29.6304) (18.5742, 29.5381) (18.4795, 29.4448) (18.3857, 29.3507) (18.2929, 29.2559) (18.2013, 29.1603) (18.1121, 29.0629) (18.0267, 28.9627) (17.9629, 28.8793) (17.918, 28.8146) (17.8894, 28.7704) (17.8755, 28.7481) knots -1 -1 -1 -1 -1 -1 -0.98571429 -0.97142857 -0.95714286 -0.94285714 -0.92857143 -0.91428571 -0.9 -0.88571429 -0.87142857 -0.85714286 -0.84285714 -0.82857143 -0.81428571 -0.8 -0.78571429 -0.77142857 -0.75714286 -0.74285714 -0.72857143 -0.71428571 -0.7 -0.68571429 -0.67142857 -0.65714286 -0.64285714 -0.62857143 -0.61428571 -0.6 -0.58571429 -0.57142857 -0.55714286 -0.54285714 -0.52857143 -0.51428571 -0.5 -0.48571429 -0.47142857 -0.45714286 -0.44285714 -0.42857143 -0.41428571 -0.4 -0.38571429 -0.37142857 -0.35714286 -0.34285714 -0.32857143 -0.31428571 -0.3 -0.28571429 -0.27142857 -0.25714286 -0.24285714 -0.22857143 -0.21428571 -0.2 -0.18571429 -0.17142857 -0.15714286 -0.14285714 -0.12857143 -0.11428571 -0.1 -0.08571429 -0.07142857 -0.05714286 -0.04285714 -0.02857143 -0.01428571 0 0 0 0 0 0
  line L15 (17.8755, 28.7481) -> (15.6601, 25.1873)
  arc A31 (13.5473, 24.6349) -> (15.6601, 25.1873) centre (14.3122, 26.026) ccw
  arc A32 (13.5473, 24.6349) -> (9.7463, 26.3708) centre (0, 0) ccw
  arc A33 (8.7801, 28.3293) -> (9.7463, 26.3708) centre (10.2966, 27.8598) ccw
  line L16 (8.7801, 28.3293) -> (10.0204, 32.3354)
  spline S16 degree 5 poles (10.0204, 32.3354) (10.0282, 32.3606) (10.0429, 32.411) (10.0624, 32.4874) (10.0835, 32.5902) (10.1034, 32.7203) (10.1186, 32.8515) (10.1309, 32.9834) (10.1417, 33.1156) (10.1514, 33.2481) (10.1599, 33.3808) (10.1668, 33.5138) (10.1716, 33.6472) (10.174, 33.781) (10.1741, 33.9152) (10.172, 34.0498) (10.1681, 34.1847) (10.1627, 34.3198) (10.1558, 34.4551) (10.1477, 34.5905) (10.1383, 34.7261) (10.1274, 34.8619) (10.115, 34.9978) (10.1011, 35.1339) (10.0858, 35.2702) (10.069, 35.4065) (10.0509, 35.543) (10.0315, 35.6796) (10.0108, 35.8163) (9.9889, 35.9531) (9.9658, 36.0899) (9.9415, 36.2268) (9.9159, 36.3638) (9.8891, 36.5008) (9.8611, 36.6378) (9.8319, 36.7749) (9.8015, 36.912) (9.77, 37.0491) (9.7374, 37.1863) (9.7036, 37.3234) (9.6688, 37.4605) (9.6328, 37.5977) (9.5957, 37.7348) (9.5576, 37.8719) (9.5184, 38.0089) (9.4781, 38.146) (9.4367, 38.283) (9.3943, 38.4199) (9.3509, 38.5568) (9.3064, 38.6937) (9.261, 38.8304) (9.2145, 38.9672) (9.167, 39.1038) (9.1185, 39.2404) (9.0689, 39.3768) (9.0185, 39.5132) (8.967, 39.6495) (8.9145, 39.7857) (8.8611, 39.9218) (8.8068, 40.0578) (8.7514, 40.1937) (8.6952, 40.3295) (8.6379, 40.4651) (8.5798, 40.6006) (8.5207, 40.736) (8.4607, 40.8712) (8.3997, 41.0064) (8.3379, 41.1413) (8.2751, 41.2761) (8.2114, 41.4108) (8.1469, 41.5453) (8.0945, 41.6528) (8.0548, 41.7333) (8.0282, 41.787) (8.0148, 41.8138) knots 0 0 0 0 0 0 0.01428571 0.02857143 0.04285714 0.05714286 0.07142857 0.08571429 0.1 0.11428571 0.12857143 0.14285714 0.15714286 0.17142857 0.18571429 0.2 0.21428571 0.22857143 0.24285714 0.25714286 0.27142857 0.28571429 0.3 0.31428571 0.32857143 0.34285714 0.35714286 0.37142857 0.38571429 0.4 0.41428571 0.42857143 0.44285714 0.45714286 0.47142857 0.48571429 0.5 0.51428571 0.52857143 0.54285714 0.55714286 0.57142857 0.58571429 0.6 0.61428571 0.62857143 0.64285714 0.65714286 0.67142857 0.68571429 0.7 0.71428571 0.72857143 0.74285714 0.75714286 0.77142857 0.78571429 0.8 0.81428571 0.82857143 0.84285714 0.85714286 0.87142857 0.88571429 0.9 0.91428571 0.92857143 0.94285714 0.95714286 0.97142857 0.98571429 1 1 1 1 1 1
  arc A34 (8.0148, 41.8138) -> (4.0902, 42.3781) centre (0, 0) ccw